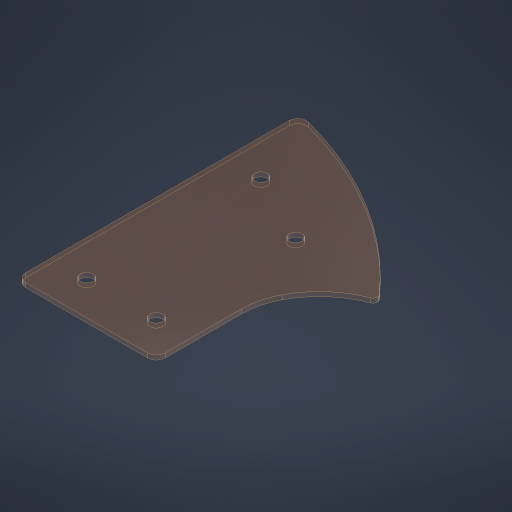
# Autodesk Inventor part: sled2
Saved by Autodesk Inventor 2024 (Build 280153000, 153)
## iProperties
Created: 2023-10-30
Part Number: sled2
Material: Polycarbonate, Smoke
Document SubType Name: Modeling
Designer: macbook
Density: 1.2 g/cm^3
Appearance: Polycarbonate - Smoked
Author: macbook
Autodesk Inventor part; units mm, degrees
ref_plane "YZ Plane" through (0, 0, 0) normal (1, 0, 0) x (0, 1, 0)
ref_plane "XZ Plane" through (0, 0, 0) normal (0, 1, 0) x (-1, 0, 0)
ref_plane "XY Plane" through (0, 0, 0) normal (0, 0, 1) x (1, 0, 0)
sketch "Sketch2" plane through (0, 0, 0) normal (0, 1, 0) x (-1, 0, 0)
  line L0 (50.8, -88.9) -> (25.4, -88.9)
  line L1 (25.4, -88.9) -> (25.4, -76.2)
  line L2 (25.4, -76.2) -> (0, -76.2)
  line L3 (50.8, -88.9) -> (50.8, -103.8965)
  line L4 (0, -76.2) -> (0, -63.5)
  line L5 (0, -63.5) -> (-22.225, -63.5)
  arc A0 (-20.6755, -65.2925) -> (46.8178, -106.9671) centre (81.3767, 24.493) ccw
  arc A1 (-20.0475, -62.76) -> (-2.9349, -47.6217) centre (-31.5353, -32.5324) ccw
  arc A2 (46.8178, -106.9671) -> (50.8, -103.8965) centre (47.625, -103.8965) ccw
  arc A3 (-20.0475, -62.76) -> (-20.6755, -65.2925) centre (-19.4836, -64.2439) ccw
  arc A4 (-2.9349, -47.6217) -> (0, -35.7694) centre (-25.4, -35.7694) ccw
  line L6 (0, -4.699) -> (47.625, -4.699)
  line L7 (50.8, -7.874) -> (50.8, -88.9)
  line L8 (0, -7.874) -> (0, -35.7694)
  line L9 (3.175, -4.699) -> (12.7, -4.699)
  line L10 (12.7, -4.699) -> (12.7, -17.399)
  line L11 (12.7, -17.399) -> (38.1, -17.399)
  line L12 (38.1, -17.399) -> (38.1, -80.899)
  line L13 (12.7, -17.399) -> (12.7, -68.199)
  arc A5 (50.8, -7.874) -> (47.625, -4.699) centre (47.625, -7.874) ccw
  arc A6 (3.175, -4.699) -> (0, -7.874) centre (3.175, -7.874) ccw
  circle A7 centre (38.1, -17.399) radius 2.3812
  circle A8 centre (12.7, -17.399) radius 2.3813
  circle A9 centre (12.7, -68.199) radius 2.3812
  circle A10 centre (38.1, -80.899) radius 2.3813
  point P0 (0, 0)
  point P1 (50.8, -107.95)
  point P2 (0, -39.6875)
  point P3 (-20.886, -63.5)
  point P4 (50.8, -4.699)
  dimension "d3" = 12.7
  dimension "d4" = 19.05
  dimension "d5" = 12.7
  dimension "d6" = 22.225
  dimension "d18" = 3.175
  dimension "d19" = 1.5875
  dimension "d20" = 25.4
  dimension "d23" = 4.699
  dimension "d24" = 12.7
  dimension "d25" = 25.4
  dimension "d26" = 63.5
  dimension "d27" = 50.8
  dimension "d28" = 3.175
  dimension "d29" = 4.7625
  dimension "d30" = 4.7625
  dimension "d31" = 4.7625
  dimension "d32" = 4.7625
  constraints: 28 end point, 18 point on circle, 11 centre point, 9 tangent, 8 coincident, 6 point on line, 5 perpendicular, 3 vertical, 2 parallel, 1 equal radius, 1 horizontal
  measures "d3" distance of L0.end L1.end
  measures "d4" distance of L0.start point (50.8, -107.95)
  measures "d5" distance of L2.end L4.end
  measures "d6" distance of L4.end L5.end
  measures "d18" radius of A2
  measures "d19" radius of A3
  measures "d20" radius of A4
  measures "d23" distance of point (0, 0) L6.start
  measures "d24" distance of L6.start L9.end
  measures "d25" distance of L10.end L11.end
  measures "d26" distance of L11.end L12.end
  measures "d27" distance of L10.end L13.end
  measures "d28" radius of A5
  measures "d29" diameter of A7
  measures "d30" diameter of A8
  measures "d31" diameter of A9
  measures "d32" diameter of A10
extrude "Extrusion1" add sketch "Sketch2" along normal blind 1.5875
body "Solid1"
